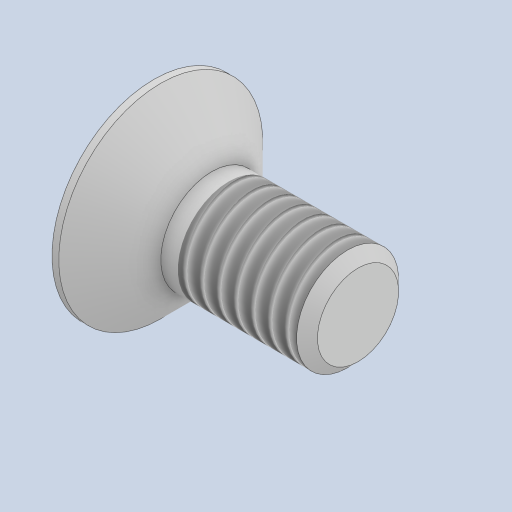
# Autodesk Inventor part: HFBCM3-6
Saved by Autodesk Inventor 2023 (Build 270158000, 158)
## iProperties
Category: PARTsolutions
Company: MISUMI
Created: 2024-12-05
Part Number: HFBCM3-6
Material: Generic
Catalog Web Link: www.cadenas.de
Description: HFBCM, SHFBS, HFBMB-Hexagon Socket Head Cap Screws for Aluminum Frames
Vendor: MISUMI
Document SubType Name: Modeling
Designer: psAdmin
Manufacturer: MISUMI
Mass: 0.0571522 g
Surface Area: 1.13814 cm^2
Volume: 0.0571522 cm^3
Density: 1 g/cm^3
Appearance: PSOLRGB-191-191-191
PSOL_IDENT_0: {$CADENAS_DATA/23d-libs/misumi/metric/38_al_extrusions_blackets/nuts/shfbs.prj},182 {VTYP=3D},{NB=HF
PSOL_IDENT_1: BCM3-6},{LINA=HFBCM3-6},{NN=HFBCM, SHFBS, HFBMB},{DATE=30.07.2021 12:55:02},{GEOMDATE=22.09.2009 00:
PSOL_IDENT_2: 00:00},{VERSION=},{LINEID=10},{WBVAR=MAT,ST,L,SET},{WBNUMERIC=L}  {NB=HFBCM3-6},{LINA=HFBCM3-6},{KT=
PSOL_IDENT_3: DUMMY},{PN=HFBCM3-6},{MAT=HFB},{MATA= 'HFB', 'SCM435(4137 Alloy Steel)(1.7220_34CrMo4)' , 'SHFB'  , '
PSOL_IDENT_4: SUS304(304 Stainless Steel)(1.4301_X5CrNi18-10)' },{ST=CM},{STA= 'CM' , 'Trivalent Chromate Plating'
PSOL_IDENT_5: , 'MB' , 'Trivalent Chromate (Black)' },{M=3},{L=6},{LL=Full Thread},{LLN=3.8},{M1=3},{LA=6,8,10,12
PSOL_IDENT_6: },{NDM=3},{KDM=2.385665},{MP=3X0.5},{A=6},{E=1.7},{B=2.0},{SET=},{SETA='', 'w/o SET1 (Set of 500pcs.
PSOL_IDENT_7: )', '-SET1'  , 'with SET1 (Set of 500pcs.)'},{P=0.50},{COLOR=0.75,0.75,0.75,0.00}
NB: HFBCM3-6
NN: HFBCM, SHFBS, HFBMB
NT: Hexagon Socket Head Cap Screws for Aluminum Frames
NBSYN: $PN.
LINA: HFBCM3-6
CATALOG: Misumi
PN: HFBCM3-6
MAT: 4137 Alloy Steel
ST: Trivalent Chromate Plating
M: 3
L: 6
LL: Full Thread
MP: 3X0.5
A: 6
E: 1.7
B: 2
SET: w/o SET1 (Set of 500pcs.)
SUPPLIER: MISUMI
ARTICLENO: HFBCM3-6
BOMINFO: HFBCM3-6
CREATOR: CADENAS GmbH
Title: HFBCM3-6
Author: Cadenas PARTsolutions
Comments: Hexagon Socket Head Cap Screws for Aluminum Frames
Autodesk Inventor part; units mm, degrees
sketch "Sketch_1" plane through (0, 0, 0) normal (0, 0, 1) x (1, 0, 0)
  line L0 (4.3, 0) -> (0, 0)
  line L1 (-1.7, 0) -> (-1.7, 3)
  line L2 (-1.7, 3) -> (-1.5, 3)
  line L3 (-1.5, 3) -> (0, 1.5)
  line L4 (0, 1.5) -> (3.9935, 1.5)
  line L5 (3.9935, 1.5) -> (4.3, 1.1935)
  line L6 (4.3, 1.1935) -> (4.3, 0)
  line L7 (4.3, 0) -> (-1.7, 0)
  constraints: 16 end point
revolve "Revolution1" add sketch "Sketch_1" angle 360 about axis through (4.3, 0, 0) along (1, 0, 0)
thread "Thread1" size "M3x0.5" class "6g" standard "ISO Metric profile" length 3.4935
sketch "Sketch2" plane through (-1.7, 0, 0) normal (-1, 0, 0) x (0, 0, 1)
  point P0 (0, 0)
hole "Hole1" at (-1.7, 0, 0) direction (1, 0, 0) diameter 2 depth 0.85 tip angle 150
sketch "Sketch_3" plane through (-1.7, 0, 0) normal (1, 0, 0) x (0, 0, -1)
  line L0 (-1, -0.5774) -> (0, -1.1547)
  line L1 (0, -1.1547) -> (1, -0.5774)
  line L2 (1, -0.5774) -> (1, 0.5774)
  line L3 (1, 0.5774) -> (0, 1.1547)
  line L4 (0, 1.1547) -> (-1, 0.5774)
  line L5 (-1, 0.5774) -> (-1, -0.5774)
  constraints: 12 end point
extrude "Extrusion1" cut sketch "Sketch_3" along normal blind 0.85
ref_plane "bolt_to_nut_XY" through (4.3, 0, 0) normal (1, 0, 0) x (0, 0, -1)
ref_plane "bolt_to_nut_YZ" through (4.3, 0, 0) normal (0, 0, -1) x (0, 1, 0)
ref_plane "bolt_to_nut_ZX" through (4.3, 0, 0) normal (0, 1, 0) x (1, 0, 0)
ref_plane "dummy_to_bolt_XY" through (0, 0, 0) normal (1, 0, 0) x (0, 0, -1)
ref_plane "dummy_to_bolt_YZ" through (0, 0, 0) normal (0, 0, -1) x (0, 1, 0)
ref_plane "dummy_to_bolt_ZX" through (0, 0, 0) normal (0, 1, 0) x (1, 0, 0)
body "Solid1"
